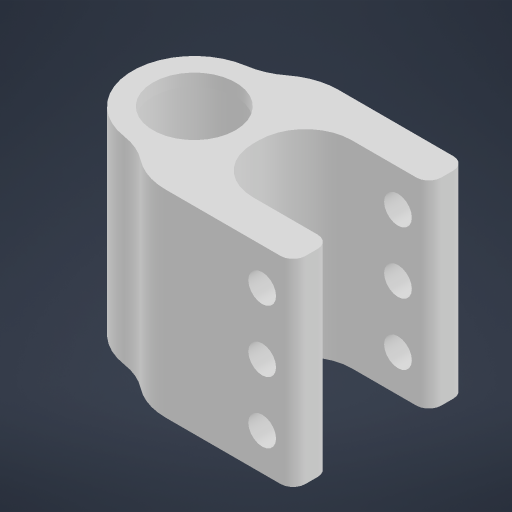
# Autodesk Inventor part: button bottom part 1
Saved by Autodesk Inventor 2024.1 (Build 281209000, 209)
## iProperties
Created: 2025-01-09
Part Number: button bottom part 1
Material: Generic
Document SubType Name: Modeling
Designer: Vibhu Iyer
Density: 1 g/cm^3
Appearance: Default
Author: Vibhu Iyer
Autodesk Inventor part; units mm, degrees
ref_plane "YZ Plane" through (0, 0, 0) normal (1, 0, 0) x (0, 1, 0)
ref_plane "XZ Plane" through (0, 0, 0) normal (0, 1, 0) x (-1, 0, 0)
ref_plane "XY Plane" through (0, 0, 0) normal (0, 0, 1) x (1, 0, 0)
sketch "Sketch1" plane through (0, 0, 0) normal (0, 1, 0) x (-1, 0, 0)
  circle A0 centre (0, 0) radius 10
  circle A1 centre (0, 0) radius 6.7
  circle A2 centre (0, 0) radius 7.7
  line L0 (-10, 8) -> (-10, -8)
  line L1 (0, 0) -> (-40.0758, 0) construction
  line L2 (-5, 8) -> (-30, 8)
  line L3 (-30, 8) -> (-30, 14)
  line L4 (-30, 14) -> (-5, 14)
  line L5 (-5, 14) -> (-5, 8)
  line L6 (-5, -8) -> (-30, -8)
  line L7 (-30, -8) -> (-30, -14)
  line L8 (-30, -14) -> (-5, -14)
  line L9 (-5, -14) -> (-5, -8)
  line L10 (0, -10) -> (-5, -11)
  line L11 (0, 10) -> (-5, 11)
  point P0 (-10, 0)
  point P1 (-10, 0)
  point P2 (2.5508, 9.6692)
  point P3 (2.5508, -9.6692)
  point P4 (-30, 11)
  point P5 (-10, 8)
  point P6 (-5, 8.6603)
  point P7 (-5, -8.6603)
  point P8 (-6, -8)
  point P9 (-6, 8)
  dimension "d0" = 13.4
  dimension "d1" = 15.4
  dimension "d37" = 20
  dimension "d38" = 20
  dimension "d39" = 6
  dimension "d40" = 5
  dimension "d46" = 16
  constraints: 24 end point, 5 midpoint, 4 point on circle, 4 symmetric about line, 3 centre point, 3 coincident, 3 horizontal, 2 parallel, 2 point on line, 2 vertical alignment, 1 horizontal alignment, 1 perpendicular, 1 tangent, 1 vertical, 1 other
  measures "d0" diameter of A1
  measures "d1" diameter of A2
  measures "d37" diameter of A0
  measures "d38" distance from line of point (-30, 11) L0
  measures "d39" distance between parallel lines of L2 L4
  measures "d40" distance between parallel lines of L0 L5
  measures "d46" distance between parallel lines of L2 L6
extrude "Extrusion1" add sketch "Sketch1" along normal blind 2 contours A0 L9 L6 L2 L5 | A0 L5 L11 | L10 L9 A0 | L5 L2 A0 | A0 L2 L3 L4 L5 | L9 L8 L7 L6 A0 | A0 L6 L9 | A0 L0 L2 | L6 L0 A0 | A2
extrude "Extrusion2" add sketch "Sketch1" against normal blind 30 contours A0 L9 L6 L2 L5 | A0 L5 L11 | L10 L9 A0 | L5 L2 A0 | A0 L2 L3 L4 L5 | L9 L8 L7 L6 A0 | A0 L6 L9 | A0 L0 L2 | L6 L0 A0
sketch "Sketch2" plane through (0, 0, 0) normal (1, 0, 0) x (0, 1, 0)
  circle A0 centre (-25, 0) radius 1.75
  line L0 (-30, -7.7) -> (-30, 7.7) projected
  point P0 (0, 0)
  dimension "d7" = 3.5
  dimension "d8" = 5
  constraints: 1 centre point, 1 horizontal alignment
  measures "d7" diameter of A0
  measures "d8" distance from line of A0.centre L0
extrude "Extrusion3" cut sketch "Sketch2" along normal mid plane 62.5
fillet "Fillet2" radius 7.5 2 edges at (10, -14, -8) (10, -14, 8)
sketch "Sketch4" plane through (29.508, -30, 14) normal (0, 0, 1) x (1, 0, 0)
  circle A0 centre (-4.508, 6) radius 2.25
  circle A1 centre (-4.508, 16) radius 2.25
  circle A2 centre (-4.508, 26) radius 2.25
  line L0 (-4.508, 6) -> (-4.508, 16) construction
  line L1 (-4.508, 16) -> (-4.508, 26) construction
  line L2 (0.492, 0) -> (0.492, 32) projected
  point P0 (-29.508, 30)
  point P1 (0.492, 16)
  point P2 (0.492, 16)
  dimension "d32" = 4.5
  dimension "d33" = 10
  dimension "d41" = 5
  constraints: 4 end point, 3 centre point, 2 equal radius, 2 horizontal alignment, 2 vertical, 1 collinear, 1 midpoint
  measures "d32" diameter of A1
  measures "d33" distance of L0.start L0.end
  measures "d41" distance between parallel lines of L1 L2
extrude "Extrusion7" cut sketch "Sketch4" against normal up to surface (28 mm away)
fillet "Fillet5" radius 10 2 edges at (5, -14, -11) (5, -14, 11)
fillet "Fillet6" radius 10 2 edges at (5, -14, -14) (5, -14, 14)
fillet "Fillet7" radius 10 2 edges at (0, -14, 10) (0, -14, -10)
fillet "Fillet4" radius 2 4 edges at (30, -14, -14) (30, -14, -8) (30, -14, 8) (30, -14, 14)
body "Solid1"
